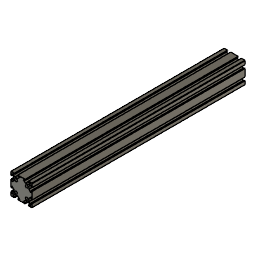
Parametric_extrusion_generator (Autodesk Fusion 360 design; units mm, degrees)
Autodesk Fusion 360 part; units mm, degrees
sketch "Sketch1" plane through (0, 0, 0) normal (0, 1, 0) x (1, 0, 0)
  line L0 (7.5, 7.5) -> (-7.5, 7.5)
  line L1 (-7.5, 7.5) -> (-7.5, -7.5)
  line L2 (-7.5, -7.5) -> (7.5, -7.5)
  line L3 (7.5, -7.5) -> (7.5, 7.5)
  line L4 (7.5, 7.5) -> (-7.5, -7.5) construction
  line L5 (-7.5, 7.5) -> (7.5, -7.5) construction
  line L6 (6, 6) -> (-6, 6)
  line L7 (-6, 6) -> (-6, -6)
  line L8 (-6, -6) -> (6, -6)
  line L9 (6, -6) -> (6, 6)
  line L10 (3, -3) -> (-3, -3)
  line L11 (-3, -3) -> (-3, 3)
  line L12 (-3, 3) -> (3, 3)
  line L13 (3, 3) -> (3, -3)
  line L14 (3, -3) -> (-3, 3) construction
  line L15 (-3, -3) -> (3, 3) construction
  circle A0 centre (0, 0) radius 1.875
  line L16 (2.25, -7.5) -> (-2.25, -7.5)
  line L17 (-2.25, -7.5) -> (-2.25, 7.5)
  line L18 (-2.25, 7.5) -> (2.25, 7.5)
  line L19 (2.25, 7.5) -> (2.25, -7.5)
  line L20 (2.25, -7.5) -> (-2.25, 7.5) construction
  line L21 (-2.25, -7.5) -> (2.25, 7.5) construction
  line L22 (7.5, 2.25) -> (-7.5, 2.25)
  line L23 (-7.5, 2.25) -> (-7.5, -2.25)
  line L24 (-7.5, -2.25) -> (7.5, -2.25)
  line L25 (7.5, -2.25) -> (7.5, 2.25)
  line L26 (7.5, 2.25) -> (-7.5, -2.25) construction
  line L27 (-7.5, 2.25) -> (7.5, -2.25) construction
  line L28 (7.5, -7.5) -> (-7.5, 7.5)
  line L29 (-7.5, 6.4393) -> (6.4393, -7.5)
  line L30 (7.5, -6.4393) -> (-6.4393, 7.5)
  line L31 (6.4393, 7.5) -> (-7.5, -6.4393)
  line L32 (-7.5, -7.5) -> (7.5, 7.5)
  line L33 (-6.4393, -7.5) -> (7.5, 6.4393)
  dimension "d3" = 15
  dimension "d4" = 15
  dimension "d7" = -1.5
  dimension "d10" = 6
  dimension "d11" = 6
  dimension "d12" = 3.75
  dimension "d13" = 4.5
  dimension "d14" = 15
  dimension "d15" = 15
  dimension "d16" = 4.5
  dimension "d17" = 0.75
  dimension "d18" = 0.75
  dimension "d19" = 0.75
  dimension "d54" = 0.75
  constraint horizontal L0
  constraint perpendicular L0 L1
  constraint parallel L0 L2
  constraint parallel L1 L3
  constraint coincident L4 A0.centre
  constraint coincident L5 A0.centre
  constraint coincident A0.centre origin
  constraint horizontal L10
  constraint perpendicular L10 L11
  constraint parallel L10 L12
  constraint parallel L11 L13
  constraint coincident L14 A0.centre
  constraint coincident L15 A0.centre
  constraint horizontal L16
  constraint perpendicular L16 L17
  constraint parallel L16 L18
  constraint parallel L17 L19
  constraint coincident L20 A0.centre
  constraint coincident L21 A0.centre
  constraint horizontal L22
  constraint perpendicular L22 L23
  constraint parallel L22 L24
  constraint parallel L23 L25
  constraint coincident L26 A0.centre
  constraint coincident L27 A0.centre
  constraint coincident L1 L31.end
  constraint coincident L0 L31.start
  constraint coincident L0 L30.end
  constraint coincident L1 L29.start
  constraint coincident L3 L30.start
  constraint coincident L2 L29.end
  constraint coincident L2 L33.start
  constraint coincident L3 L33.end
  measures "d3" distance of L1.end L2.end
  measures "d4" distance of L0.end L1.end
  measures "d10" distance of L11.end L12.end
  measures "d11" distance of L10.end L11.end
  measures "d12" diameter of A0
  measures "d13" distance of L17.end L18.end
  measures "d14" distance of L16.end L17.end
  measures "d15" distance of L23.end L24.end
  measures "d16" distance of L22.end L23.end
sketch "Sketch3" plane through (0, 0, 0) normal (0, 1, 0) x (1, 0, 0)
  line L0 (-7.5, 7.5) -> (-7.5, -7.5)
  line L1 (-7.5, -7.5) -> (7.5, -7.5)
  line L2 (-7.5, -7.5) -> (22.5, -7.5)
  line L3 (22.5, -7.5) -> (22.5, 22.5)
  line L4 (22.5, 22.5) -> (-7.5, 22.5)
  line L5 (-7.5, 22.5) -> (-7.5, -7.5)
  dimension "d30" = 30
  dimension "d31" = 30
  constraint horizontal L2
  constraint vertical L3
  constraint horizontal L4
  constraint vertical L5
  constraint coincident L0.end L1.start
  measures "d30" distance of L0.end L2.end
  measures "d31" distance of L0.end L4.end
extrude "Extrude3" add sketch "Sketch3" along normal blind 300
extrude "Extrude4" cut sketch "Sketch1" along normal blind 300 contours L2 L8 L16 L17 L19 | L8 L19 L29 | L8 L10 L17 L19 L29 L33 | L8 L17 L33
extrude "Extrude5" cut sketch "Sketch1" along normal blind 300 contours L1 L7 L22 L23 L24 | L7 L22 L29 | L7 L11 L22 L24 L29 L31 | L7 L24 L31
extrude "Extrude6" cut sketch "Sketch1" along normal blind 300 contours A0 L30 L31 L32 | A0 L30 L32 L33 | A0 L30 L33 | A0 L30 L31 | L28 L30 L31 L32 | L28 L30 L32 L33 | A0 L28 L30 L33 | A0 L28 L30 L31 | L28 L29 L31 L32 | L28 L29 L32 L33 | A0 L28 L29 L33 | A0 L28 L29 L31 | A0 L29 L31 L32 | A0 L29 L32 L33 | A0 L29 L33 | A0 L29 L31
pattern_linear "R-Pattern1" count 2 spacing 15 along (1, 0, 0) of "Extrude4"
pattern_linear "R-Pattern2" count 2 spacing 15 along (0, 0, -1) of "Extrude5"
pattern_linear "R-Pattern3" count 2 spacing 15 along (0, 0, -1) count 2 spacing 15 along (1, 0, 0) of "Extrude6"
ref_plane "WorkPlane1" through (7.5, 150, -7.5) normal (1, 0, 0) x (0, 0, -1)
ref_plane "WorkPlane2" through (7.5, 150, -7.5) normal (0, 0, 1) x (1, 0, 0)
pattern_circular "C-Pattern1" count 2 over 360 about axis through (7.5, 66, -7.5) along (0, 1, 0) of "Extrude4", "Extrude5", "R-Pattern1", "R-Pattern2"
fillet "Fillet1" radius 0.375 4 edges at (-7.5, 150, 7.5) (22.5, 150, 7.5) (22.5, 150, -22.5) (-7.5, 150, -22.5)
equation "extrusionWidth = extrusionHeight"
equation "extrusionHeight = 15 mm"
equation "d3 = extrusionHeight"
equation "d4 = extrusionHeight"
equation "d7 = -0.1 * extrusionHeight"
equation "width = 2"
equation "height = 2"
equation "d10 = 0.4 * extrusionHeight"
equation "d11 = 0.4 * extrusionHeight"
equation "d12 = 0.25 * extrusionHeight"
equation "d13 = 0.3 * extrusionHeight"
equation "d14 = extrusionHeight"
equation "d15 = extrusionHeight"
equation "d16 = 0.3 * extrusionHeight"
equation "d17 = 0.05 * extrusionHeight"
equation "d18 = 0.05 * extrusionHeight"
equation "d19 = 0.05 * extrusionHeight"
equation "extrudsionLength = 300 mm"
equation "d30 = extrusionHeight * width"
equation "d31 = extrusionHeight * height"
equation "d32 = extrudsionLength"
equation "d34 = extrudsionLength"
equation "d36 = extrudsionLength"
equation "d38 = extrudsionLength"
equation "d40 = width"
equation "d42 = extrusionHeight"
equation "d44 = height"
equation "d46 = -extrusionHeight"
equation "d48 = height"
equation "d49 = width"
equation "d50 = -extrusionHeight"
equation "d51 = extrusionHeight"
equation "d54 = 0.05 * extrusionHeight"
equation "d56 = 0.025 * extrusionHeight"
